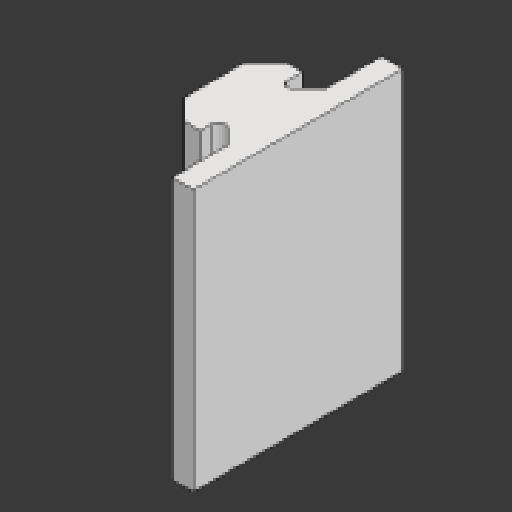
# Autodesk Inventor part: LED Mount
Saved by Autodesk Inventor 2023 (Build 270158000, 158)
## iProperties
Created: 2023-01-06
Part Number: LED Mount
Material: Generic
Document SubType Name: Modeling
Designer: alber
Density: 1 g/cm^3
Appearance: Default
Author: alber
Autodesk Inventor part; units mm, degrees
ref_plane "YZ Plane" through (0, 0, 0) normal (1, 0, 0) x (0, 1, 0)
ref_plane "XZ Plane" through (0, 0, 0) normal (0, 1, 0) x (-1, 0, 0)
ref_plane "XY Plane" through (0, 0, 0) normal (0, 0, 1) x (1, 0, 0)
sketch "Sketch1" plane through (0, 0, 0) normal (0, 1, 0) x (-1, 0, 0)
  line L0 (-10.3707, 15.395) -> (-8.7381, 17.0275)
  arc A0 (-7.8549, 16.6) -> (-8.7381, 17.0275) centre (-8.4, 16.6) ccw
  line L1 (-7.8549, 16.6) -> (-7.8549, 15.135)
  line L2 (-7.8549, 15.135) -> (-6.3429, 15.135)
  line L3 (-6.3429, 15.135) -> (-4.3451, 17.1329)
  line L4 (-4.3451, 17.1329) -> (-4.3451, 22.8671)
  line L5 (-4.3451, 22.8671) -> (-6.3429, 24.865)
  line L6 (-6.3429, 24.865) -> (-7.8549, 24.865)
  line L7 (-7.8549, 24.865) -> (-7.8549, 23.8568)
  arc A1 (-9.0499, 23.3618) -> (-7.8549, 23.8568) centre (-8.5549, 23.8568) ccw
  line L8 (-9.0499, 23.3618) -> (-10.3707, 24.6827)
  line L9 (-10.3707, 15.395) -> (-10.3707, 10.0707)
  line L10 (-10.3707, 10.0707) -> (-12.399, 10.0707)
  line L11 (-10.3707, 10.0707) -> (-18.3707, 10.0707)
  line L12 (-18.3707, 10.0707) -> (-18.3707, 50.0707)
  line L13 (-18.3707, 50.0707) -> (-14.3707, 50.0707)
  line L14 (-10.3707, 15.395) -> (-10.3707, 10.0707)
  line L15 (-14.3707, 50.0707) -> (-14.3707, 28.6827)
  line L16 (-14.3707, 28.6827) -> (-10.3707, 24.6827)
  line L17 (-10.3707, 24.6827) -> (-10.3707, 24.865)
  line L18 (-10.3707, 50.0707) -> (-10.3707, 28.8927)
  line L19 (-10.3707, 24.865) -> (-10.3707, 24.6827)
  point P0 (0, 0)
  point P1 (-9.0499, 23.3618)
  dimension "d5" = 40
  constraints: 40 end point, 4 parallel, 4 point on circle, 3 point on line, 2 centre point, 2 horizontal, 2 vertical, 1 perpendicular
  measures "d5" distance of L11.end L12.end
extrude "Extrusion1" add sketch "Sketch1" along normal blind 25
sketch "Sketch3" plane through (10.3707, 0, 10.0707) normal (0, 0, -1) x (-1, 0, 0)
  point P0 (10.3707, 0)
fillet "Fillet1" radius 3 1 edges at (18.3707, 12.5, 10.0707)
fillet "Fillet2" radius 3 1 edges at (18.3707, 12.5, 50.0707)
body "Solid1"
